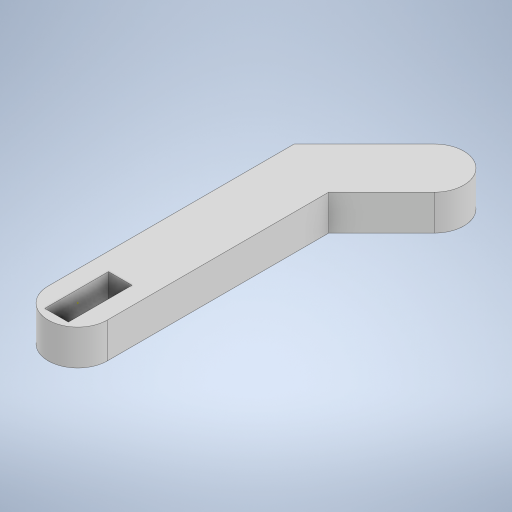
# Autodesk Inventor part: Arm 1
Saved by Autodesk Inventor 2023 (Build 270158000, 158)
## iProperties
Created: 2024-06-27
Part Number: Arm 1
Material: Generic
Document SubType Name: Modeling
Designer: Swoby
Density: 1 g/cm^3
Appearance: Default
Author: Swoby
Autodesk Inventor part; units mm, degrees
ref_plane "YZ Plane" through (0, 0, 0) normal (1, 0, 0) x (0, 1, 0)
ref_plane "XZ Plane" through (0, 0, 0) normal (0, 1, 0) x (-1, 0, 0)
ref_plane "XY Plane" through (0, 0, 0) normal (0, 0, 1) x (1, 0, 0)
sketch "Sketch1" plane through (0, 0, 0) normal (0, 1, 0) x (-1, 0, 0)
  circle A0 centre (0, 0) radius 25
  line L0 (25, 0) -> (25, -208.3553)
  line L1 (25, -208.3553) -> (-34.3223, -267.6777)
  line L2 (-25, 0) -> (-25, -187.6447)
  line L3 (-25, -187.6447) -> (-69.6777, -232.3223)
  circle A1 centre (-52, -250) radius 25
  dimension "d0" = 50
  dimension "d1" = 50
  dimension "d2" = 250
  dimension "d3" = 27
  dimension "d4" = 135
  constraints: 8 end point, 4 point on circle, 4 tangent, 2 centre point, 2 parallel, 1 coincident, 1 vertical
  measures "d0" diameter of A0
  measures "d1" diameter of A1
  measures "d2" vertical distance of point (0, 0) A1.centre
  measures "d3" distance from line of L2 A1.centre
  measures "d4" angle of L1 L0
extrude "Extrusion1" add sketch "Sketch1" along normal blind 30
sketch "Sketch2" plane through (0, 0, 0) normal (0, -1, 0) x (1, 0, 0)
  line L0 (-10, -36) -> (10, -36)
  line L1 (10, -36) -> (10, 18)
  line L2 (10, 18) -> (-10, 18)
  line L3 (-10, 18) -> (-10, -36)
  line L4 (-10, -29) -> (10, -29)
  line L5 (10, -29) -> (10, 11)
  line L6 (10, 11) -> (-10, 11)
  line L7 (-10, 11) -> (-10, -29)
  point P0 (0, 0)
  point P1 (-10, 11)
  dimension "d7" = 54
  dimension "d8" = 20
  dimension "d9" = 10
  dimension "d10" = 7
  dimension "d11" = 40
  dimension "d12" = 36
  constraints: 16 end point, 4 parallel, 2 horizontal, 2 perpendicular, 2 point on line
  measures "d7" distance of L2.end L0.start
  measures "d8" distance of L1.end L2.end
  measures "d9" distance from line of point (0, 0) L3
  measures "d10" distance between parallel lines of L2 L6
  measures "d11" distance between parallel lines of L4 L6
  measures "d12" distance from line of L0 point (0, 0)
extrude "Extrusion2" cut sketch "Sketch2" against normal through all contours L3 L6 L1 L4
sketch "Sketch3" plane through (0, 30, 0) normal (0, 1, 0) x (1, 0, 0)
  line L0 (-10, -18) -> (10, -18)
  line L1 (10, -18) -> (10, 36)
  line L2 (10, 36) -> (-10, 36)
  line L3 (-10, 36) -> (-10, -18)
  line L4 (10, -11) -> (-10, -11) projected
  line L5 (-10, 29) -> (10, 29) projected
  point P0 (0, 0)
  dimension "d15" = 7
  dimension "d16" = 7
  constraints: 8 end point, 2 parallel, 2 point on line, 1 horizontal, 1 perpendicular
  measures "d15" distance between parallel lines of L2 L5
  measures "d16" distance between parallel lines of L0 L4
extrude "Extrusion3" cut sketch "Sketch3" against normal blind 21 contours L3 L4 L1 L0 | L3 L2 L1 L5
sketch "Sketch4" plane through (0, 30, 0) normal (0, 1, 0) x (1, 0, 0)
  point P0 (0, 0)
body "Solid1"
